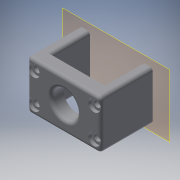
# Autodesk Inventor part: Upper_bearing_support_outside
Saved by Autodesk Inventor 2019.3 (Build 233278000, 278)
## iProperties
Created: 2020-09-08
Part Number: Upper_bearing_support_outside
Material: Generisch
Document SubType Name: Modeling
Designer: Nicolas Frick
Density: 1 g/cm^3
Appearance: Vorgabe
Author: Nicolas Frick
Autodesk Inventor part; units mm, degrees
ref_plane "YZ Plane" through (0, 0, 0) normal (1, 0, 0) x (0, 1, 0)
ref_plane "XZ Plane" through (0, 0, 0) normal (0, 1, 0) x (-1, 0, 0)
sketch "Skizze1" plane through (0, 0, 0) normal (0, 0, 1) x (1, 0, 0)
  circle A0 centre (0, 0) radius 8 construction
  line L0 (-30, -17.5) -> (30, -17.5) construction
  line L1 (30, -17.5) -> (30, 17.5) construction
  line L2 (30, 17.5) -> (-30, 17.5) construction
  line L3 (-30, 17.5) -> (-30, -17.5) construction
  circle A1 centre (0, 0) radius 9 construction
  circle A2 centre (0, 0) radius 14 construction
  line L4 (-15, -15) -> (15, -15)
  line L5 (15, 15) -> (-15, 15)
  line L6 (-15, -15) -> (15, 15) construction
  line L7 (15, -15) -> (-15, 15) construction
  line L8 (-22.5, -15) -> (22.5, -15)
  line L9 (22.5, -15) -> (22.5, 15)
  line L10 (22.5, 15) -> (-22.5, 15)
  line L11 (-22.5, 15) -> (-22.5, -15)
  line L12 (-22.5, -15) -> (22.5, 15) construction
  line L13 (22.5, -15) -> (-22.5, 15) construction
  circle A3 centre (0, 0) radius 8
  point P0 (0, 0)
  constraints: 20 end point, 4 midpoint, 3 parallel, 2 horizontal, 1 centre point, 1 coincident, 1 concentric, 1 perpendicular
extrude "Extrusion1" add sketch "Skizze1" along normal blind 32
ref_plane "Arbeitsebene1" through (0, 0, 0) normal (0, 0, 1) x (1, 0, 0)
sketch "Skizze2" plane through (0, 0, 0) normal (0, 0, 1) x (1, 0, 0)
  circle A0 centre (0, 0) radius 13.8 construction
  circle A1 centre (0, 0) radius 14 construction
  line L0 (22.5, 15) -> (-22.5, 15) construction
  line L1 (22.5, -15) -> (22.5, 15) construction
  line L2 (-22.5, -15) -> (22.5, -15) construction
  line L3 (-22.5, 15) -> (-22.5, -15) construction
  line L4 (-22.5, -15) -> (22.5, -15) projected
  line L5 (-16, 15) -> (16, 15)
  line L6 (16, 15) -> (16, -15)
  line L7 (16, -15) -> (-16, -15)
  line L8 (-16, -15) -> (-16, 15)
  line L9 (-16, 15) -> (16, -15) construction
  line L10 (16, 15) -> (-16, -15) construction
  point P0 (0, 0)
  dimension "d5" = 32
  constraints: 12 end point, 2 midpoint, 2 parallel, 1 horizontal, 1 perpendicular, 1 point on line
  measures "d5" distance of L6.end L7.end
ref_plane "Arbeitsebene2" through (-7.2804, -7.2804, 24.15) normal (0, 0, -1) x (-0.0257355, 0.9996688, 0)
extrude "Extrusion2" cut sketch "Skizze2" along normal up to surface (24.15 mm away)
sketch "Skizze3" plane through (0, 0, 32) normal (0, 0, 1) x (1, 0, 0)
  circle A0 centre (0, 0) radius 8 construction
  line L0 (-22.5, -15) -> (22.5, -15) construction
  line L1 (22.5, -15) -> (22.5, 15) construction
  line L2 (22.5, 15) -> (-22.5, 15) construction
  line L3 (-22.5, 15) -> (-22.5, -15) construction
  line L4 (16, -15) -> (16, 15) construction
  line L5 (-16, 15) -> (-16, -15) construction
  line L6 (22.5, -11.8361) -> (18.5, -11.8361) construction
  line L7 (16, -15) -> (22.5, -15) construction
  line L8 (18.5, -15) -> (18.5, -9) construction
  line L9 (22.5, 15) -> (-22.5, 15) construction
  line L10 (18.5, 15) -> (18.5, 9) construction
  line L11 (-22.5, 15) -> (-22.5, -15) construction
  line L12 (-22.5, -9) -> (-18.4855, -9) construction
  line L13 (-22.5, 9) -> (-18.4855, 9) construction
  point P0 (0, 0)
  dimension "d9" = 4
  dimension "d10" = 6
  dimension "d11" = 6
  constraints: 10 end point, 5 perpendicular, 5 point on line, 4 coincident
  measures "d9" distance of L6.start L6.end
  measures "d10" distance of L8.start L8.end
  measures "d11" distance of L10.start L10.end
hole "Bohrung1" at (18.5, -9, 32) at (18.5, 9, 32) at (-18.4855, -9, 32) at (-18.4855, 9, 32) direction (0, 0, -1) diameter 4.2 end through all counterbore diameter 7.2 counterbore depth 2
fillet "Rundung1" radius 2 4 edges at (0, -15, 32) (22.5, 0, 32) (0, 15, 32) (-22.5, 0, 32)
fillet "Rundung2" radius 2 1 edges at (-8, 0, 32)
fillet "Rundung3" radius 2 12 edges at (21.9142, 14.4142, 31.4142) (22.5, 15, 15) (16, 15, 12.075) (-16, 15, 12.075) (-21.9142, 14.4142, 31.4142) (-22.5, 15, 15) (21.9142, -14.4142, 31.4142) (22.5, -15, 15) (-21.9142, -14.4142, 31.4142) (-22.5, -15, 15) (-16, -15, 12.075) (16, -15, 12.075)
